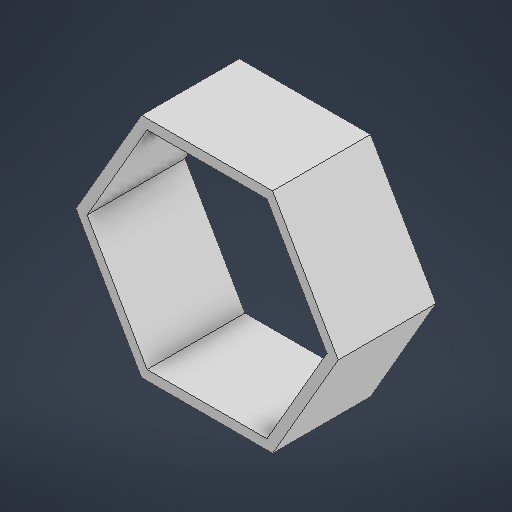
# Autodesk Inventor part: tolerance_test
Saved by Autodesk Inventor 2026.2 (Build 302298000, 298)
## iProperties
Created: 2026-04-15
Part Number: tolerance_test
Material: Generic
Document SubType Name: Modeling
Designer: cbast
Density: 1 g/cm^3
Appearance: Default
Author: cbast
## iProperties of the stored document tolerance_test_3DPrint.ipt
Created: 2026-04-15
Part Number: tolerance_test_3DPrint
Material: Generic
Document SubType Name: Modeling
Designer: cbast
Density: 1 g/cm^3
Appearance: Default
Author: cbast
Autodesk Inventor part; units mm, degrees
ref_plane "YZ Plane" through (0, 0, 0) normal (1, 0, 0) x (0, 1, 0)
ref_plane "XZ Plane" through (0, 0, 0) normal (0, 1, 0) x (-1, 0, 0)
ref_plane "XY Plane" through (0, 0, 0) normal (0, 0, 1) x (1, 0, 0)
sketch "Sketch1" plane through (0, 0, 0) normal (0, 0, 1) x (1, 0, 0)
  line L0 (0, 0) -> (17.0068, 0) construction
  line L1 (-3.0599, 5.2999) -> (-6.1198, 0)
  line L2 (-6.1198, 0) -> (-3.0599, -5.2999)
  line L3 (-3.0599, -5.2999) -> (3.0599, -5.2999)
  line L4 (3.0599, -5.2999) -> (6.1198, 0)
  line L5 (6.1198, 0) -> (3.0599, 5.2999)
  line L6 (3.0599, 5.2999) -> (-3.0599, 5.2999)
  line L7 (-6.6971, 0) -> (-3.3486, 5.7999)
  line L8 (-3.3486, 5.7999) -> (3.3486, 5.7999)
  line L9 (3.3486, 5.7999) -> (6.6971, 0)
  line L10 (6.6971, 0) -> (3.3486, -5.7999)
  line L11 (3.3486, -5.7999) -> (-3.3486, -5.7999)
  line L12 (-3.3486, -5.7999) -> (-6.6971, 0)
  point P0 (5.7734, 0)
  dimension "d7" = 0.5
  constraints: 26 end point, 1 horizontal, 1 point on line, 5 other
  measures "d7" distance between parallel lines of L1 L7
extrude "Extrusion1" add sketch "Sketch1" along normal blind 5
body "Solid1"
